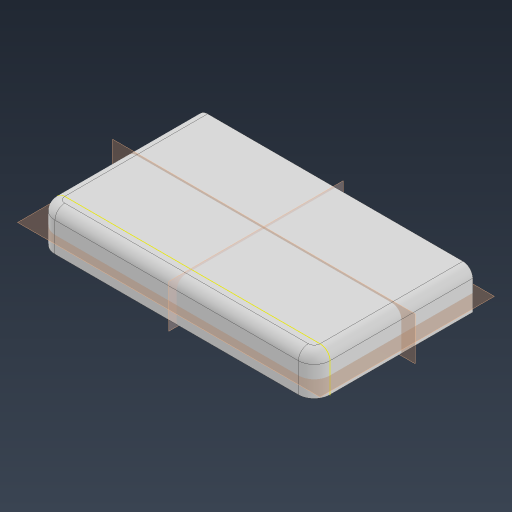
# Autodesk Inventor part: Крышка_электроники
Saved by Autodesk Inventor 2023.2 (Build 272271030, 271C)
## iProperties
Created: 2025-12-29
Part Number: Крышка_электроники
Material: Типовые
Document SubType Name: Modeling
Designer: Олег Коноваленко
Density: 1 g/cm^3
Appearance: По умолчанию
Author: Олег Коноваленко
Autodesk Inventor part; units mm, degrees
sketch "Эскиз1" plane through (0, 0, 0) normal (0, 0, 1) x (1, 0, 0)
  line L0 (-70, -8.5) -> (-70, 11.5)
  line L1 (-70, 11.5) -> (70, 11.5)
  line L2 (70, 11.5) -> (70, -8.5)
  line L3 (70, -8.5) -> (67, -8.5)
  line L4 (67, -8.5) -> (67, 8.5)
  line L5 (67, 8.5) -> (-67, 8.5)
  line L6 (-67, 8.5) -> (-67, -8.5)
  line L7 (-67, -8.5) -> (-70, -8.5)
  line L8 (0, 15.5) -> (0, -12.5) construction
  line L9 (-98, 0) -> (98, 0) projected
  circle A0 centre (62, 3.5) radius 5
  circle A1 centre (65, 6.5) radius 5
  circle A2 centre (-65, 6.5) radius 5
  circle A3 centre (-62, 3.5) radius 5
  point P0 (0, 0)
  point P1 (0, 11.5)
  point P2 (-67, 0)
  point P3 (62, 8.5)
  point P4 (67, 3.5)
  point P5 (70, 6.5)
  point P6 (65, 11.5)
  point P7 (-67, 3.5)
  point P8 (-62, 8.5)
  point P9 (-65, 11.5)
  point P10 (-70, 6.5)
  dimension "d0" = 134
  dimension "d2" = 3
  dimension "d3" = 3
  dimension "d4" = 20
  dimension "d8" = 10
  constraints: 16 end point, 8 tangent, 6 perpendicular, 4 centre point, 3 equal radius, 2 equal length, 2 midpoint, 2 point on line, 1 parallel, 1 vertical
  measures "d0" distance between parallel lines of L4 L6
  measures "d2" distance between parallel lines of L5 L1
  measures "d3" distance between parallel lines of L2 L4
  measures "d4" distance of L0.start L0.end
  measures "d8" diameter of A0
extrude "Выдавливание1" add sketch "Эскиз1" along normal mid plane 72.75 contours L0 L9 L6 L7 | L0 A2 L6 L9 | A2 L5 L6 | L1 A1 L5 A2 | A1 L4 L5 | L6 L5 A3 | L2 L9 L4 A1 | L2 L3 L4 L9 | L5 L4 A0
sketch "Эскиз3" plane through (0, 0, 36.375) normal (0, 0, 1) x (1, 0, 0)
  arc A0 (67, 3.5) -> (62, 8.5) centre (62, 3.5) ccw projected
  line L0 (62, 8.5) -> (62, 11.5)
  line L1 (65, 11.5) -> (-65, 11.5) projected
  arc A1 (70, 6.5) -> (65, 11.5) centre (65, 6.5) ccw projected
  line L2 (70, -8.5) -> (70, 6.5) projected
  line L3 (67, -8.5) -> (70, -8.5) projected
  line L4 (67, 3.5) -> (67, -8.5) projected
  arc A2 (-62, 8.5) -> (-67, 3.5) centre (-62, 3.5) ccw projected
  line L5 (-67, -8.5) -> (-67, 3.5) projected
  line L6 (-70, -8.5) -> (-67, -8.5) projected
  line L7 (-70, 6.5) -> (-70, -8.5) projected
  arc A3 (-65, 11.5) -> (-70, 6.5) centre (-65, 6.5) ccw projected
  line L8 (-62, 8.5) -> (62, 8.5) projected
  line L9 (-62, 8.5) -> (-62, 11.5)
  point P0 (0, 0)
  constraints: 4 end point, 2 point on line, 2 vertical
revolve "Вращение1" add sketch "Эскиз3" angle 90 about axis through (-62, 8.5, 36.375) along (0, 1, 0) contours A2 L5 L6 L7 A3 L1 L9
revolve "Вращение2" add sketch "Эскиз3" angle 90 about axis through (62, 8.5, 36.375) along (0, -1, 0) contours A0 L0 L1 A1 L2 L3 L4
sketch "Эскиз4" plane through (62, 8.5, 36.375) normal (-1, 0, 0) x (0, 0, 1)
  line L0 (3, 3) -> (0, 3) projected
  line L1 (0, 0) -> (0, 3) projected
  arc A0 (5, -5) -> (0, 0) centre (0, -5) ccw projected
  line L2 (5, -5) -> (5, -17) projected
  line L3 (5, -17) -> (8, -17) projected
  line L4 (8, -17) -> (8, -2) projected
  arc A1 (8, -2) -> (3, 3) centre (3, -2) ccw projected
  point P0 (-36.375, -8.5)
extrude "Выдавливание2" add sketch "Эскиз4" along normal up to surface (124 mm away)
